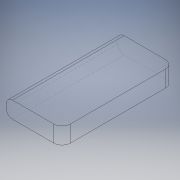
# Autodesk Inventor part: Onn-USB-Hub
Saved by Autodesk Inventor 2017 (Build 210142000, 142)
## iProperties
Created: 2018-04-08
Part Number: Onn-USB-Hub
Material: Generic
Document SubType Name: Modeling
Designer: MtgSaber
Density: 1 g/cm^3
Appearance: Default
Author: MtgSaber
Autodesk Inventor part; units mm, degrees
ref_plane "YZ Plane" through (0, 0, 0) normal (1, 0, 0) x (0, 1, 0)
ref_plane "XZ Plane" through (0, 0, 0) normal (0, 1, 0) x (-1, 0, 0)
ref_plane "XY Plane" through (0, 0, 0) normal (0, 0, 1) x (1, 0, 0)
sketch "Sketch1" plane through (0, 0, 0) normal (0, 1, 0) x (-1, 0, 0)
  line L0 (21.4313, 42.8625) -> (-21.4313, 42.8625)
  line L1 (-21.4313, 42.8625) -> (-21.4313, -42.8625)
  line L2 (-21.4313, -42.8625) -> (21.4312, -42.8625)
  line L3 (21.4312, -42.8625) -> (21.4313, 42.8625)
  line L4 (0, -60.0075) -> (0, 60.0075) construction
  line L5 (30.0038, 0) -> (-30.0038, 0) construction
  point P0 (0, 0)
  point P1 (0, -42.8625)
  point P2 (-21.4313, 0)
  dimension "d0" = 85.725
  dimension "d1" = 42.8625
  constraints: 8 end point, 2 midpoint, 2 parallel, 2 point on line, 1 horizontal, 1 perpendicular
  measures "d0" distance of L0.end L1.end
  measures "d1" distance of L1.end L2.end
extrude "Extrusion1" add sketch "Sketch1" along normal blind 12.7
fillet "Fillet1" radius 4.7625 2 edges at (-21.4312, 12.7, 0) (-21.4312, 0, 0)
fillet "Fillet2" radius 6.35 2 edges at (21.4313, 6.35, 42.8625) (21.4313, 6.35, -42.8625)
body "Solid1"
